Autodesk Inventor part; units mm, degrees
(part 2 of 2)
sketch "Sketch22" plane through (0, 0, 0) normal (0, 0, -1) x (-1, 0, 0)
  circle A0 centre (435.0722, 321.6304) radius 3.2639 projected
  circle A1 centre (198.3647, 418.811) radius 2.5119 projected
  circle A2 centre (440.3741, 420.236) radius 2.1989 projected
  circle A3 centre (542.5208, 420.236) radius 2.1989 projected
  circle A4 centre (644.6428, 420.236) radius 2.1989 projected
  circle A5 centre (491.4414, 357.8965) radius 2.1989 projected
  circle A6 centre (593.5881, 357.8965) radius 2.1989 projected
  circle A7 centre (398.5657, 358.1076) radius 2.1723 projected
  circle A8 centre (500.7124, 358.1076) radius 2.1723 projected
  circle A9 centre (602.8344, 358.1076) radius 2.1723 projected
  circle A10 centre (449.633, 420.0249) radius 2.1723 projected
  circle A11 centre (551.7797, 420.0249) radius 2.1723 projected
  circle A12 centre (644.6222, 194.6304) radius 3.2639 projected
  circle A13 centre (57.15, 98.044) radius 2.4116 projected
  circle A14 centre (197.0948, 59.563) radius 2.4116 projected
  circle A15 centre (542.5208, 158.3585) radius 2.1989 projected
  circle A16 centre (491.4414, 158.3585) radius 2.1989 projected
  circle A17 centre (440.3741, 96.019) radius 2.1989 projected
  circle A18 centre (542.5208, 96.019) radius 2.1989 projected
  circle A19 centre (644.6428, 96.019) radius 2.1989 projected
  circle A20 centre (449.633, 96.2301) radius 2.1723 projected
  circle A21 centre (500.7124, 96.2301) radius 2.1723 projected
  circle A22 centre (398.5657, 158.1474) radius 2.1723 projected
  circle A23 centre (500.7124, 158.1474) radius 2.1723 projected
  circle A24 centre (602.8344, 158.1474) radius 2.1723 projected
  circle A25 centre (551.7797, 158.1474) radius 2.1723 projected
  circle A26 centre (449.633, 158.1474) radius 2.1723 projected
  circle A27 centre (398.5657, 96.2301) radius 2.1723 projected
  circle A28 centre (551.7797, 96.2301) radius 2.1723 projected
  circle A29 centre (602.8344, 96.2301) radius 2.1723 projected
  circle A30 centre (593.5881, 96.019) radius 2.1989 projected
  circle A31 centre (491.4414, 96.019) radius 2.1989 projected
  circle A32 centre (593.5881, 158.3585) radius 2.1989 projected
  circle A33 centre (440.3741, 158.3585) radius 2.1989 projected
  circle A34 centre (644.6428, 158.3585) radius 2.1989 projected
  circle A35 centre (197.0948, 95.631) radius 2.4116 projected
  circle A36 centre (57.15, 57.15) radius 2.4116 projected
  circle A37 centre (435.0722, 194.6304) radius 3.2639 projected
  circle A38 centre (602.8344, 420.0249) radius 2.1723 projected
  circle A39 centre (500.7124, 420.0249) radius 2.1723 projected
  circle A40 centre (398.5657, 420.0249) radius 2.1723 projected
  circle A41 centre (551.7797, 358.1076) radius 2.1723 projected
  circle A42 centre (449.633, 358.1076) radius 2.1723 projected
  circle A43 centre (644.6428, 357.8965) radius 2.1989 projected
  circle A44 centre (542.5208, 357.8965) radius 2.1989 projected
  circle A45 centre (440.3741, 357.8965) radius 2.1989 projected
  circle A46 centre (593.5881, 420.236) radius 2.1989 projected
  circle A47 centre (491.4414, 420.236) radius 2.1989 projected
  circle A48 centre (151.1207, 418.811) radius 2.5119 projected
  circle A49 centre (644.6222, 321.6304) radius 3.2639 projected
  circle A50 centre (12.7, 486.7275) radius 2.0701 projected
  circle A51 centre (12.7, 461.3275) radius 2.0701 projected
  circle A52 centre (12.7, 435.9275) radius 2.0701 projected
  circle A53 centre (12.7, 410.5275) radius 2.0701 projected
  circle A54 centre (12.7, 385.1275) radius 2.0701 projected
  circle A55 centre (12.7, 359.7275) radius 2.0701 projected
  circle A56 centre (12.7, 334.3275) radius 2.0701 projected
  circle A57 centre (12.7, 308.9275) radius 2.0701 projected
  circle A58 centre (12.7, 283.5275) radius 2.0701 projected
  circle A59 centre (12.7, 258.1275) radius 2.0701 projected
  circle A60 centre (12.7, 232.7275) radius 2.0701 projected
  circle A61 centre (12.7, 207.3275) radius 2.0701 projected
  circle A62 centre (12.7, 181.9275) radius 2.0701 projected
  circle A63 centre (12.7, 156.5275) radius 2.0701 projected
  circle A64 centre (12.7, 131.1275) radius 2.0701 projected
  circle A65 centre (12.7, 105.7275) radius 2.0701 projected
  circle A66 centre (12.7, 80.3275) radius 2.0701 projected
  circle A67 centre (12.7, 54.9275) radius 2.0701 projected
  circle A68 centre (12.7, 29.5275) radius 2.0701 projected
  circle A69 centre (673.1, 486.7275) radius 2.0701 projected
  circle A70 centre (673.1, 461.3275) radius 2.0701 projected
  circle A71 centre (673.1, 435.9275) radius 2.0701 projected
  circle A72 centre (673.1, 410.5275) radius 2.0701 projected
  circle A73 centre (673.1, 385.1275) radius 2.0701 projected
  circle A74 centre (673.1, 359.7275) radius 2.0701 projected
  circle A75 centre (673.1, 334.3275) radius 2.0701 projected
  circle A76 centre (673.1, 308.9275) radius 2.0701 projected
  circle A77 centre (673.1, 283.5275) radius 2.0701 projected
  circle A78 centre (673.1, 258.1275) radius 2.0701 projected
  circle A79 centre (673.1, 232.7275) radius 2.0701 projected
  circle A80 centre (673.1, 207.3275) radius 2.0701 projected
  circle A81 centre (673.1, 181.9275) radius 2.0701 projected
  circle A82 centre (673.1, 156.5275) radius 2.0701 projected
  circle A83 centre (673.1, 131.1275) radius 2.0701 projected
  circle A84 centre (673.1, 105.7275) radius 2.0701 projected
  circle A85 centre (673.1, 80.3275) radius 2.0701 projected
  circle A86 centre (673.1, 54.9275) radius 2.0701 projected
  circle A87 centre (673.1, 29.5275) radius 2.0701 projected
  line L0 (252.73, 332.105) -> (252.73, 490.855) projected
  line L1 (252.73, 490.855) -> (392.43, 490.855) projected
  line L2 (392.43, 490.855) -> (392.43, 332.105) projected
  line L3 (392.43, 332.105) -> (252.73, 332.105) projected
  line L4 (392.43, 25.4) -> (252.73, 25.4) projected
  line L5 (252.73, 25.4) -> (252.73, 184.15) projected
  line L6 (252.73, 184.15) -> (392.43, 184.15) projected
  line L7 (392.43, 184.15) -> (392.43, 25.4) projected
  circle A88 centre (12.7, 503.555) radius 2.0828 projected
  circle A89 centre (12.7, 12.7) radius 2.0828 projected
  circle A90 centre (38.1, 503.555) radius 2.0828 projected
  circle A91 centre (38.1, 12.7) radius 2.0828 projected
  circle A92 centre (63.5, 503.555) radius 2.0828 projected
  circle A93 centre (63.5, 12.7) radius 2.0828 projected
  circle A94 centre (88.9, 503.555) radius 2.0828 projected
  circle A95 centre (88.9, 12.7) radius 2.0828 projected
  circle A96 centre (114.3, 503.555) radius 2.0828 projected
  circle A97 centre (114.3, 12.7) radius 2.0828 projected
  circle A98 centre (139.7, 503.555) radius 2.0828 projected
  circle A99 centre (139.7, 12.7) radius 2.0828 projected
  circle A100 centre (165.1, 503.555) radius 2.0828 projected
  circle A101 centre (165.1, 12.7) radius 2.0828 projected
  circle A102 centre (190.5, 503.555) radius 2.0828 projected
  circle A103 centre (190.5, 12.7) radius 2.0828 projected
  circle A104 centre (215.9, 503.555) radius 2.0828 projected
  circle A105 centre (215.9, 12.7) radius 2.0828 projected
  circle A106 centre (241.3, 503.555) radius 2.0828 projected
  circle A107 centre (241.3, 12.7) radius 2.0828 projected
  circle A108 centre (266.7, 503.555) radius 2.0828 projected
  circle A109 centre (266.7, 12.7) radius 2.0828 projected
  circle A110 centre (292.1, 503.555) radius 2.0828 projected
  circle A111 centre (292.1, 12.7) radius 2.0828 projected
  circle A112 centre (317.5, 503.555) radius 2.0828 projected
  circle A113 centre (317.5, 12.7) radius 2.0828 projected
  circle A114 centre (342.9, 503.555) radius 2.0828 projected
  circle A115 centre (342.9, 12.7) radius 2.0828 projected
  circle A116 centre (368.3, 503.555) radius 2.0828 projected
  circle A117 centre (368.3, 12.7) radius 2.0828 projected
  circle A118 centre (393.7, 503.555) radius 2.0828 projected
  circle A119 centre (393.7, 12.7) radius 2.0828 projected
  circle A120 centre (419.1, 503.555) radius 2.0828 projected
  circle A121 centre (419.1, 12.7) radius 2.0828 projected
  circle A122 centre (444.5, 503.555) radius 2.0828 projected
  circle A123 centre (444.5, 12.7) radius 2.0828 projected
  circle A124 centre (469.9, 503.555) radius 2.0828 projected
  circle A125 centre (469.9, 12.7) radius 2.0828 projected
  circle A126 centre (495.3, 503.555) radius 2.0828 projected
  circle A127 centre (495.3, 12.7) radius 2.0828 projected
  circle A128 centre (520.7, 503.555) radius 2.0828 projected
  circle A129 centre (520.7, 12.7) radius 2.0828 projected
  circle A130 centre (546.1, 503.555) radius 2.0828 projected
  circle A131 centre (546.1, 12.7) radius 2.0828 projected
  circle A132 centre (571.5, 503.555) radius 2.0828 projected
  circle A133 centre (571.5, 12.7) radius 2.0828 projected
  circle A134 centre (596.9, 503.555) radius 2.0828 projected
  circle A135 centre (596.9, 12.7) radius 2.0828 projected
  circle A136 centre (622.3, 503.555) radius 2.0828 projected
  circle A137 centre (622.3, 12.7) radius 2.0828 projected
  circle A138 centre (647.7, 503.555) radius 2.0828 projected
  circle A139 centre (647.7, 12.7) radius 2.0828 projected
  circle A140 centre (673.1, 503.555) radius 2.0828 projected
  circle A141 centre (673.1, 12.7) radius 2.0828 projected
  line L8 (0, 0) -> (685.8, 0) projected
  line L9 (685.8, 0) -> (685.8, 516.255) projected
  line L10 (685.8, 516.255) -> (0, 516.255) projected
  line L11 (0, 516.255) -> (0, 0) projected
fillet "Corner Round1" radius 6.35 12 edges at (0, 516.255, 0.7937) (-685.8, 516.255, 0.7937) (-685.8, 0, 0.7937) (0, 0, 0.7937) (-392.43, 184.15, 0.7937) (-252.73, 184.15, 0.7937) (-392.43, 25.4, 0.7937) (-252.73, 25.4, 0.7937) (-392.43, 332.105, 0.7937) (-392.43, 490.855, 0.7937) (-252.73, 332.105, 0.7937) (-252.73, 490.855, 0.7937)
sketch "Sketch24" plane through (0, 0, 0) normal (0, 0, -1) x (-1, 0, 0)
  line L0 (25.4, 25.4) -> (660.4, 25.4) projected
  line L1 (660.4, 602.615) -> (660.4, -86.36) projected
  line L2 (628.5069, 25.4) -> (628.5069, 97.991)
  line L3 (660.4, 97.991) -> (620.522, 97.991)
  line L4 (620.522, 97.991) -> (620.522, 156.157)
  circle A0 centre (620.522, 156.157) radius 2.1717
  circle A1 centre (620.522, 97.991) radius 2.1717
  point P0 (0, 0)
  dimension "d133" = 72.591
  dimension "d134" = 39.878
  dimension "d135" = 58.166
  dimension "d136" = 4.3434
  dimension "d137" = 4.3434
  constraints: 6 end point, 2 centre point, 2 coincident, 2 perpendicular, 2 point on line, 1 parallel
  measures "d133" distance of L2.start L2.end
  measures "d134" distance of L3.start L3.end
  measures "d135" distance of L3.end L4.end
  measures "d136" diameter of A0
  measures "d137" diameter of A1
extrude "Cut11" cut sketch "Sketch24" against normal blind 1.5875 contours A1 L4 L3 | L3 L4 A1 | A0
ref_plane "Work Plane1" through (-679.45, 258.1275, 0) normal (0, -1, 0) x (1, 0, 0)
mirror "Mirror1" about plane through (-679.45, 258.1275, 0) normal (0, -1, 0) of "Cut11"
extrude "Cut12" cut sketch "Sketch17" against normal blind 1.5875 contours A300 | A301
sketch "Sketch25" plane through (0, 0, 0) normal (0, 0, -1) x (-1, 0, 0)
  circle A0 centre (198.3647, 418.811) radius 2.5119 projected
  circle A1 centre (151.1207, 418.811) radius 2.5119 projected
  circle A2 centre (151.1207, 418.811) radius 12.7
  circle A3 centre (198.3647, 418.811) radius 12.7
  point P0 (0, 0)
  dimension "d147" = 25.4
  dimension "d148" = 25.4
  constraints: 2 centre point, 2 coincident
  measures "d147" diameter of A2
  measures "d148" diameter of A3
extrude "Cut13" cut sketch "Sketch25" against normal blind 1.5875
equation "\"d17\" = Thickness"
equation "\"d65\" = Thickness"
equation "\"BendRadius\" = Thickness"
equation "\"BendReliefWidth\" = Thickness"
equation "\"BendReliefDepth\" = 0.5 * Thickness"
equation "\"CornerReliefSize\" = 4 * Thickness"
equation "\"MinimumRemnant\" = 2 * Thickness"
equation "\"TransitionRadius\" = BendRadius"
equation "\"JacobiRadiusSize\" = Thickness"
equation "\"GapSize\" = Thickness"
equation "\"d2\" = BendRadius"
equation "\"Thickness\" = 1.5875"
body "Solid1"
